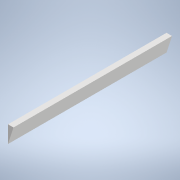
# Autodesk Inventor part: degrau
Saved by Autodesk Inventor 2020 (Build 240168000, 168)
## iProperties
Created: 2020-04-24
Part Number: degrau
Material: Genérico
Document SubType Name: Modeling
Designer: gi-se
Density: 1 g/cm^3
Appearance: Padrão
Author: gi-se
Autodesk Inventor part; units mm, degrees
ref_plane "YZ Plane" through (0, 0, 0) normal (1, 0, 0) x (0, 1, 0)
ref_plane "XZ Plane" through (0, 0, 0) normal (0, 1, 0) x (-1, 0, 0)
ref_plane "XY Plane" through (0, 0, 0) normal (0, 0, 1) x (1, 0, 0)
sketch "Esboço1" plane through (0, 0, 0) normal (0, 0, 1) x (1, 0, 0)
  line L0 (2.5785, 54.25) -> (22.6, 54.25) projected
  arc A0 (30, 46.85) -> (22.6, 54.25) centre (22.6, 46.85) ccw projected
  line L1 (-4.9941, -1.6438) -> (-12.1764, -3.5683) projected
  line L2 (-27, -22.8868) -> (-27, -54.25) projected
  line L3 (-27, -54.25) -> (-30, -54.25) projected
  line L4 (-30, -54.25) -> (-30, 1.15) projected
  line L5 (-25, 6.15) -> (-14.8, 6.15) projected
  arc A1 (-14.8, 6.15) -> (-11.2, 9.75) centre (-14.8, 9.75) ccw projected
  line L6 (-11.2, 9.75) -> (-11.2, 44.0112) projected
  line L7 (-8.7623, 48.3048) -> (0.0162, 53.5436) projected
  circle A2 centre (22.6, 46.85) radius 0.8 projected
  line L8 (-22, -38.7498) -> (-27, -38.7498)
  line L9 (-27, -38.7498) -> (-27, -54.25)
  line L10 (-27, -54.25) -> (-22, -38.7498)
  arc A3 (-25, 6.15) -> (-30, 1.15) centre (-25, 1.15) ccw projected
  arc A4 (-8.7623, 48.3048) -> (-11.2, 44.0112) centre (-6.2, 44.0112) ccw projected
  arc A5 (2.5785, 54.25) -> (0.0162, 53.5436) centre (2.5785, 49.25) ccw projected
  arc A6 (-12.1764, -3.5683) -> (-27, -22.8868) centre (-7, -22.8868) ccw projected
  line L11 (30, -54.25) -> (19.6, -54.25) projected
  line L12 (19.6, -54.25) -> (19.6, -22.8868) projected
  arc A7 (19.6, -22.8868) -> (4.7764, -3.5683) centre (-0.4, -22.8868) ccw projected
  line L13 (4.7764, -3.5683) -> (-2.4059, -1.6438) projected
  arc A8 (-2.4059, -1.6438) -> (-4.9941, -1.6438) centre (-3.7, -6.4734) ccw projected
  line L14 (30, 46.85) -> (30, -54.25) projected
  point P0 (0, 0)
  constraints: 6 end point
extrude "Extrusão1" add sketch "Esboço1" against normal blind 144 contours L2 L8 L10
